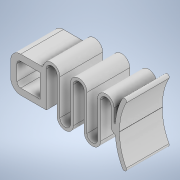
# Autodesk Inventor part: resortePlano0.8mmX3mmD
Saved by Autodesk Inventor 2021.5 (Build 255421000, 421)
## iProperties
Created: 2024-11-30
Part Number: resortePlano0.8mmX3mmD
Material: Genérico
Document SubType Name: Modeling
Designer: Joho_
Density: 1 g/cm^3
Appearance: Valor por defecto
Author: Joho_
Autodesk Inventor part; units mm, degrees
ref_plane "YZ Plane" through (0, 0, 0) normal (1, 0, 0) x (0, 1, 0)
ref_plane "XZ Plane" through (0, 0, 0) normal (0, 1, 0) x (-1, 0, 0)
ref_plane "XY Plane" through (0, 0, 0) normal (0, 0, 1) x (1, 0, 0)
sketch "Boceto1" plane through (0, 0, 0) normal (0, 0, 1) x (1, 0, 0)
  line L0 (3, -11.4) -> (3, -5.5)
  line L1 (3, -5.5) -> (-2.2, -5.5)
  arc A0 (-5.5, -2.2) -> (-2.2, -5.5) centre (-2.2, -2.2) ccw
  line L2 (-5.5, -2.2) -> (-5.5, 2.2)
  arc A1 (-2.2, 5.5) -> (-5.5, 2.2) centre (-2.2, 2.2) ccw
  line L3 (-2.2, 5.5) -> (3, 5.5)
  line L4 (3, 5.5) -> (3, 11.4)
  line L5 (3, 3) -> (-2.2, 3)
  arc A2 (-2.2, 3) -> (-3, 2.2) centre (-2.2, 2.2) ccw
  line L6 (-3, 2.2) -> (-3, -2.2)
  arc A3 (-3, -2.2) -> (-2.2, -3) centre (-2.2, -2.2) ccw
  line L7 (-2.2, -3) -> (3, -3)
  line L8 (3, -3) -> (3, 3)
  line L9 (-2.2, 3.25) -> (3.25, 3.25)
  line L10 (3.25, 3.25) -> (3.25, -3.25)
  line L11 (3.25, -3.25) -> (-2.2, -3.25)
  arc A4 (-3.25, -2.2) -> (-2.2, -3.25) centre (-2.2, -2.2) ccw
  line L12 (-3.25, -2.2) -> (-3.25, 2.2)
  arc A5 (-2.2, 3.25) -> (-3.25, 2.2) centre (-2.2, 2.2) ccw
  line L13 (-2.2, 5) -> (5, 5)
  line L14 (5, 5) -> (5, -5)
  line L15 (5, -5) -> (-2.2, -5)
  arc A6 (-5, -2.2) -> (-2.2, -5) centre (-2.2, -2.2) ccw
  line L16 (-5, -2.2) -> (-5, 2.2)
  arc A7 (-2.2, 5) -> (-5, 2.2) centre (-2.2, 2.2) ccw
  line L17 (5, 0) -> (23, 0)
  line L18 (5, 5) -> (6.5, 5)
  line L19 (8.8007, 5) -> (8.0007, 5)
  line L20 (8.0007, 5) -> (8.0007, -5)
  line L21 (8.0007, -5) -> (8.8007, -5)
  line L22 (8.8007, -5) -> (8.8007, 5)
  line L23 (8.8007, -5) -> (10.3007, -5)
  line L24 (12.6007, -5) -> (11.8007, -5)
  line L25 (11.8007, -5) -> (11.8007, 5)
  line L26 (11.8007, 5) -> (12.6007, 5)
  line L27 (12.6007, 5) -> (12.6007, -5)
  arc A8 (8.8007, -5) -> (11.8007, -5) centre (10.3007, -5) ccw
  arc A9 (8.0007, -5) -> (12.6007, -5) centre (10.3007, -5) ccw
  arc A10 (8.0007, 5) -> (4.9993, 5) centre (6.5, 5) ccw
  arc A11 (8.8007, 5) -> (4.1993, 5) centre (6.5, 5) ccw
  line L28 (16.4021, 5) -> (15.6021, 5)
  line L29 (15.6021, 5) -> (15.6021, -5)
  line L30 (15.6021, -5) -> (16.4021, -5)
  line L31 (16.4021, -5) -> (16.4021, 5)
  line L32 (20.2021, -5) -> (19.4021, -5)
  line L33 (19.4021, -5) -> (19.4021, 5)
  line L34 (19.4021, 5) -> (20.2021, 5)
  line L35 (20.2021, 5) -> (20.2021, -5)
  arc A12 (16.4021, -5) -> (19.4021, -5) centre (17.9021, -5) ccw
  arc A13 (15.6021, -5) -> (20.2021, -5) centre (17.9021, -5) ccw
  arc A14 (15.6021, 5) -> (12.6007, 5) centre (14.1014, 5) ccw
  arc A15 (16.4021, 5) -> (11.8007, 5) centre (14.1014, 5) ccw
  line L36 (24.0036, 5) -> (23.2036, 5)
  line L37 (23.2036, 5) -> (23.2036, -0.2574)
  line L38 (23.2036, -5) -> (24.0036, -5)
  line L39 (24.0036, -1.1409) -> (24.0036, 5)
  arc A16 (23.2036, 5) -> (20.2021, 5) centre (21.7028, 5) ccw
  arc A17 (24.0036, 5) -> (19.4021, 5) centre (21.7028, 5) ccw
  arc A18 (26.3756, 8.5) -> (24.3756, 0) centre (41.5966, 0.4333) ccw
  circle A19 centre (24.3756, 0) radius 1.2
  arc A20 (27.4359, 7.9381) -> (25.5752, 0.0302) centre (41.5966, 0.4333) ccw
  line L40 (25.6, 8.5) -> (25.9736, 8.302)
  arc A21 (27.4359, 7.9381) -> (26.3756, 8.5) centre (26.9058, 8.219) ccw
  arc A22 (24.3756, 0) -> (26.3756, -8.5) centre (41.5966, -0.4333) ccw
  arc A23 (26.3756, -8.5) -> (27.4359, -7.9381) centre (26.9058, -8.219) ccw
  line L41 (26.7492, -8.302) -> (27.4359, -7.9381)
  arc A24 (25.5752, -0.0302) -> (27.4359, -7.9381) centre (41.5966, -0.4333) ccw
  line L42 (23.2036, 0) -> (24.0036, 0)
  point P0 (0, 0)
  point P1 (5, -5)
  point P2 (4.2, -5)
  point P3 (3.8, 5)
  point P4 (25.5036, -5)
  point P5 (22.4, 0)
  point P6 (24.3872, 1.1999)
  point P7 (24.0036, 1.1409)
  point P8 (23.2036, 0.2574)
  point P9 (24.3872, -1.1999)
  point P10 (25.5752, -0.0302)
  point P11 (25.5752, 0.0302)
  dimension "d1" = 0.25
  dimension "d2" = 2
  dimension "d42" = 18
  dimension "d43" = 1.5
  dimension "d45" = 0.8
  dimension "d46" = 10
  dimension "d47" = 1.5
  dimension "d48" = 0.8
  dimension "d49" = 10
  dimension "d50" = 0.8
  dimension "d51" = 10
  dimension "d52" = 1.5
  dimension "d53" = 0.8
  dimension "d54" = 10
  dimension "d55" = 0.8
  dimension "d56" = 10
  dimension "d57" = 1.5
  dimension "d62" = 1.2
  constraints: 86 end point, 51 point on circle, 28 centre point, 10 parallel, 8 horizontal, 7 coincident, 6 point on line, 5 perpendicular, 1 midpoint
  measures "d1" distance between parallel lines of L5 L9
  measures "d2" distance between parallel lines of L5 L13
  measures "d42" distance of L17.start L17.end
  measures "d43" distance of L13.end L18.end
  measures "d45" distance of L21.end L20.end
  measures "d46" distance of L20.end L19.end
  measures "d47" distance of L21.end L23.end
  measures "d48" distance of L26.end L25.end
  measures "d49" distance of L25.end L24.end
  measures "d50" distance of L31.start L29.end
  measures "d51" distance of L29.end L28.end
  measures "d52" distance of L31.start point (17.902, -5)
  measures "d53" distance of L34.end L34.start
  measures "d54" distance of L34.start L33.start
  measures "d55" distance of L38.end L38.start
  measures "d56" distance of L38.start L36.end
  measures "d57" distance of L38.end point (25.504, -5)
  measures "d62" radial gap between concentric circles of A18 A20
extrude "Extrusión1" add sketch "Boceto1" along normal blind 12 contours L13 L14 L15 A6 L16 A7 | A11 L19 A10 L13 | L22 L17 L20 L19 | L22 L21 L20 L17 | L25 L26 L27 L17 | L17 L27 L24 L25 | A8 L24 A9 L21 | A15 L28 A14 L26 | L29 L28 L31 L17 | L17 L31 L30 L29 | L30 A12 L32 A13 | L33 L34 L35 L17 | L17 L35 L32 L33 | A17 L36 A16 L34 | L39 A19 L37 L36 | A19 A18 A22 L39 | L39 L42 L37 A19 | L37 A19 | L39 A19 L37 L42 | A19 A22 A18 | A18 A21 A20 A19 | A19 A24 A23 A22
fillet "Empalme1" radius 0.8 2 edges at (4.1993, 5, 6) (24.3872, -1.1999, 6)
fillet "Empalme1" radius 0.2 2 edges at (24.0036, 1.1409, 6) (24.3872, 1.1999, 6)
